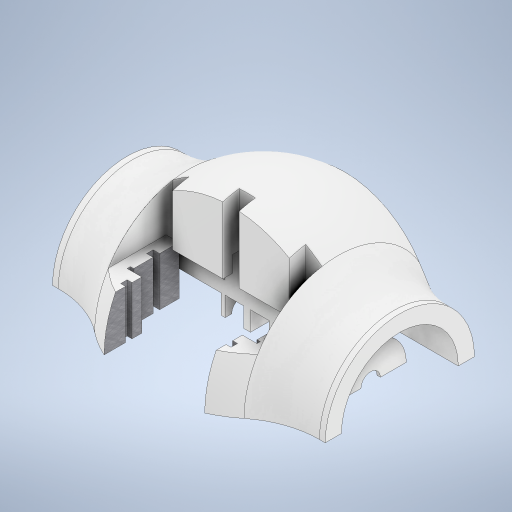
# Autodesk Inventor part: back moter middle tire lemon shape
Saved by Autodesk Inventor 2023 (Build 270158000, 158)
## iProperties
Created: 2022-10-08
Part Number: back moter middle tire lemon shape
Material: ABS プラスチック
Document SubType Name: Modeling
Designer: ellie
Density: 1.06 g/cm^3
Appearance: 積雪
Author: ellie
Autodesk Inventor part; units mm, degrees
ref_plane "YZ Plane" through (0, 0, 0) normal (1, 0, 0) x (0, 1, 0)
ref_plane "XZ Plane" through (0, 0, 0) normal (0, 1, 0) x (-1, 0, 0)
ref_plane "XY Plane" through (0, 0, 0) normal (0, 0, 1) x (1, 0, 0)
sketch "スケッチ1" plane through (0, 0, 0) normal (0, 1, 0) x (-1, 0, 0)
  circle A0 centre (0, 0) radius 37
  line L0 (0, 0) -> (0, -37)
  line L1 (0, 0) -> (0, 37)
  dimension "d0" = 74
  constraints: 4 end point, 2 point on circle, 2 vertical, 1 centre point, 1 coincident
  measures "d0" diameter of A0
revolve "回転1" add sketch "スケッチ1" angle 180 about axis through (0, 0, 0) along (0, 0, 1) picked at (-2.7444, -24.3574) contours L1 L0 A0
sketch "スケッチ5" plane through (0, 0, 0) normal (0, -1, 0) x (1, 0, 0)
  line L0 (-20, -21) -> (20, -21)
  line L1 (20, -21) -> (20, -11)
  line L2 (20, -11) -> (-20, -11)
  line L3 (-20, -11) -> (-20, -21)
  line L4 (-20, -13) -> (-20, -11)
  line L5 (0, 27) -> (-17, 27)
  line L6 (-17, 27) -> (-17, 25)
  line L7 (-17, 25) -> (0, 25)
  line L8 (0, 25) -> (0, 27)
  line L9 (0, 22) -> (-20, 22)
  line L10 (-20, 22) -> (-20, 21)
  line L11 (-20, 21) -> (0, 21)
  line L12 (0, 21) -> (0, 22)
  line L13 (0, 15) -> (-21, 15)
  line L14 (-21, 15) -> (-21, 13)
  line L15 (-21, 13) -> (0, 13)
  line L16 (0, 13) -> (0, 15)
  line L17 (0, 7) -> (-23, 7)
  line L18 (-23, 7) -> (-23, 5)
  line L19 (-23, 5) -> (0, 5)
  line L20 (0, 5) -> (0, 7)
  circle A0 centre (0, 0) radius 37 projected
  circle A1 centre (0, 0) radius 37 projected
  line L21 (0, 37) -> (0, -37)
  line L22 (37, 0) -> (-37, 0)
  line L23 (-32, 5) -> (-23, 5)
  line L24 (-23, 5) -> (-23, -5)
  line L25 (-23, -5) -> (-32, -5)
  line L26 (-32, -5) -> (-32, 5)
  line L27 (-23, -8.0262) -> (-23, 5)
  line L28 (-29, 22.9783) -> (-29, -22.9783)
  line L29 (-15.5, 27) -> (0, 27)
  line L30 (0, 27) -> (0, 37)
  line L31 (0, 37) -> (-15.5, 37)
  line L32 (-15.5, 37) -> (-15.5, 27)
  line L33 (-15.5, 25) -> (0, 25)
  line L34 (0, 25) -> (0, 22)
  line L35 (0, 22) -> (-15.5, 22)
  line L36 (-15.5, 22) -> (-15.5, 25)
  line L37 (-19, 15) -> (0, 15)
  line L38 (0, 15) -> (0, 21)
  line L39 (0, 21) -> (-19, 21)
  line L40 (-19, 21) -> (-19, 15)
  line L41 (-19, 13) -> (0, 13)
  line L42 (0, 13) -> (0, 7)
  line L43 (0, 7) -> (-19, 7)
  line L44 (-19, 7) -> (-19, 13)
  line L45 (-23, 0) -> (-39.6865, 0)
  line L46 (-23, 0) -> (-7.8337, 0)
  line L47 (-8, 5) -> (-23, 5)
  line L48 (-23, 5) -> (-23, -5)
  line L49 (-23, -5) -> (-8, -5)
  line L50 (-8, -5) -> (-8, 5)
  line L51 (-8, 5) -> (-23, -5) construction
  line L52 (-23, 5) -> (-8, -5) construction
  line L53 (-23, 7) -> (-33, 7)
  line L54 (-33, 7) -> (-33, -7)
  line L55 (-33, -7) -> (-23, -7)
  line L56 (-23, -7) -> (-23, 7)
  line L57 (-23, 7) -> (-33, -7) construction
  line L58 (-33, 7) -> (-23, -7) construction
  line L59 (-8, 5) -> (-1, 5)
  line L60 (-1, 5) -> (-1, -5)
  line L61 (-1, -5) -> (-8, -5)
  line L62 (-8, -5) -> (-8, 5)
  line L63 (-8, 5) -> (-1, -5) construction
  line L64 (-1, 5) -> (-8, -5) construction
  line L65 (-23, 5) -> (-29, 5)
  line L66 (-23, -5) -> (-29, -5)
  line L67 (-23, 7) -> (-29, 7)
  line L68 (-23, -7) -> (-29, -7)
  line L69 (27.2764, -25) -> (-27.2764, -25)
  line L70 (-8, 5) -> (-6.8, 5)
  line L71 (-6.8, 5) -> (-6.8, -5)
  line L72 (-6.8, -5) -> (-8, -5)
  line L73 (-8, -5) -> (-8, 5)
  line L74 (-3, 7) -> (0, 7)
  line L75 (0, 22) -> (-4, 22)
  line L76 (-4, 21) -> (0, 21)
  line L77 (0, 21) -> (0, 22)
  line L78 (-6, 7) -> (-1, 7)
  line L79 (-1, 5) -> (-6, 5)
  point P0 (0, -21)
  point P1 (0, -11)
  point P2 (0, 26)
  point P3 (0, 21.5)
  point P4 (0, 14)
  point P5 (0, 6)
  point P6 (-20, -16)
  point P7 (-27, -0.5262)
  point P8 (-29, -5)
  point P9 (-15.5, 23.5)
  point P10 (-15.5, 33.5969)
  point P11 (0, 27)
  point P12 (0, 25)
  point P13 (0, 13)
  point P14 (0, 15)
  point P15 (-29, 0)
  point P16 (-32, 0)
  point P17 (-23, 0)
  point P18 (-15.5, 0)
  point P19 (-28, 0)
  point P20 (-4.5, 0)
  point P21 (-8, -5)
  point P22 (-8, 5)
  point P23 (-27, 0.5)
  point P24 (-28, 0.4738)
  point P25 (-28, -11.5262)
  point P26 (-27, -11.5)
  point P27 (-23, -5)
  point P28 (-23, 5)
  point P29 (-23, 5)
  point P30 (-23, -5)
  point P31 (-8, 0)
  point P32 (-1, 0)
  point P33 (0, 21)
  point P34 (0, 22)
  point P35 (-29, -7)
  point P36 (-29, 7)
  dimension "d12" = 40
  dimension "d13" = 10
  dimension "d23" = 17
  dimension "d24" = 2
  dimension "d27" = 20
  dimension "d28" = 1
  dimension "d30" = 21
  dimension "d31" = 2
  dimension "d33" = 2
  dimension "d88" = 0
  dimension "d89" = 0
  dimension "d90" = 16
  dimension "d92" = 20
  dimension "d93" = 10
  dimension "d97" = 9
  dimension "d98" = 10
  dimension "d113" = 29
  dimension "d122" = 15.5
  dimension "d123" = 37
  dimension "d124" = 3
  dimension "d125" = 15.5
  dimension "d126" = 6
  dimension "d127" = 6
  dimension "d128" = 19
  dimension "d129" = 19
  dimension "d147" = 10
  dimension "d149" = 8
  dimension "d151" = 15
  dimension "d161" = 14
  dimension "d162" = 10
  dimension "d164" = 10
  dimension "d165" = 7
  dimension "d170" = 25
  dimension "d175" = 1.2
  dimension "d207" = 0
  constraints: 158 end point, 31 parallel, 20 horizontal, 17 perpendicular, 16 point on line, 15 midpoint, 10 collinear, 1 vertical, 20 other
  measures "d12" distance of L2.end L1.end
  measures "d13" distance of L1.end L0.end
  measures "d23" distance of L7.end L6.end
  measures "d24" distance of L6.end L5.end
  measures "d27" distance of L11.end L10.end
  measures "d28" distance of L10.end L9.end
  measures "d30" distance of L15.end L14.end
  measures "d31" distance of L14.end L13.end
  measures "d33" distance of L18.end L17.end
  measures "d89" distance from line of point (0, 0) L22
  measures "d90" distance from line of L0 point (0, -37)
  measures "d92" distance of the line from the sketch origin of L3
  measures "d93" distance from line of L5 point (0, 37)
  measures "d97" distance of L24.end L25.end
  measures "d98" distance of L23.end L24.end
  measures "d113" distance of the line from the sketch origin of L28
  measures "d122" distance of the line from the sketch origin of L32
  measures "d123" distance between parallel lines of L31 L22
  measures "d124" distance of L33.end L34.end
  measures "d126" distance of L38.end L37.end
  measures "d127" distance of L41.end L42.end
  measures "d128" distance of the line from the sketch origin of L44
  measures "d129" distance of the line from the sketch origin of L40
  measures "d147" distance of L48.end L47.end
  measures "d149" distance of the line from the sketch origin of L50
  measures "d151" distance between parallel lines of L50 L24
  measures "d161" distance between parallel lines of L55 L53
  measures "d162" distance between parallel lines of L48 L54
  measures "d164" distance between parallel lines of L61 L59
  measures "d165" distance between parallel lines of L50 L60
  measures "d170" distance between parallel lines of L69 L22
  measures "d175" distance of L71.end L72.end
  measures "d207" distance between parallel lines of L47 L19
extrude "GNSボード" cut sketch "スケッチ5" against normal blind 16 contours L8 L7 L6 L5
extrude "GNSボード止めるよう" cut sketch "スケッチ5" against normal blind 15 contours L21 L5 L32 A0 | L21 L9 L36 L7
extrude "アルミ板１" cut sketch "スケッチ5" against normal blind 20 contours L11 L10 L9 L12
extrude "メイン基板" cut sketch "スケッチ5" against normal blind 21 contours L15 L14 L13 L16
extrude "メイン止めるよう" cut sketch "スケッチ5" against normal blind 15 contours L17 L44 L15 L21 | L13 L40 L11 L21
extrude "アルミ板２" cut sketch "スケッチ5" against normal blind 20 contours L19 L18 L17 L20
extrude "電池ボックス入れ" cut sketch "スケッチ5" against normal blind 13 contours L3 L2 L21 L0 | L21 L2 L1 L0
extrude "side ut" cut sketch "スケッチ5" against normal blind 100 contours A0 L22 L54 L55 L28 | A0 L28 L53 L54 L22 | L55 L54 L22 L26 L25 L28 | L54 L53 L28 L23 L26 L22 | L25 L26 L22 L28 | L26 L23 L28 L22
extrude "motor case" add sketch "スケッチ5" against normal blind 7 contours L55 L54 L22 L26 L25 L28 | L28 L25 L27 L55 | L54 L53 L28 L23 L26 L22 | L28 L22 L24 L25 | L25 L26 L22 L28 | L50 L49 L24 L22 | L22 L24 L19 L50 | L53 L18 L23 L28 | L26 L23 L28 L22 | L28 L23 L24 L22
extrude "bottom cut" cut sketch "スケッチ5" against normal blind 90 contours L69 A0 L21 | L21 A0 L69
extrude "motor" cut sketch "スケッチ5" against normal blind 6 contours L60 L61 L71 L22 | L22 L71 L19 L60 | L71 L61 L50 L22 | L22 L50 L19 L71 | L28 L22 L24 L25 | L25 L26 L22 L28 | L50 L49 L24 L22 | L22 L24 L19 L50 | L26 L23 L28 L22 | L28 L23 L24 L22
extrude "motor block" add sketch "スケッチ5" against normal blind 10 contours L71 L61 L50 L22 | L22 L50 L19 L71
sketch "スケッチ27" plane through (-33, 0, -7) normal (-1, 0, 0) x (0, 0, 1)
  line L0 (14, 0) -> (0, 0) projected
  circle A0 centre (7, 0) radius 3
  point P0 (7, 0)
  dimension "d198" = 6
  constraints: 1 centre point, 1 midpoint
  measures "d198" diameter of A0
extrude "moter shaft" cut sketch "スケッチ27" against normal blind 27
mirror "ミラー13" about plane through (0, 0, 0) normal (1, 0, 0) of "メイン止めるよう", "メイン基板", "アルミ板１", "GNSボード止めるよう", "GNSボード", "アルミ板２", "motor", "motor case", "moter shaft", "電池ボックス入れ", "side ut", "motor block"
ref_plane "作業平面5" through (-17, 17.5, 25) normal (0, -1, 0) x (1, 0, 0)
ref_plane "作業平面6" through (20, 13, -11) normal (0, 0, -1) x (1, 0, 0)
ref_plane "作業平面7" through (29, 35, 7) normal (0, -1, 0) x (1, 0, 0)
sketch "スケッチ41" plane through (-17, 0, 25) normal (0, -1, 0) x (1, 0, 0)
  line L0 (-16, -22) -> (-15, -22) projected
  line L1 (-15, -22) -> (-15, -20) projected
  line L2 (-15, -20) -> (-6, -20) projected
  line L3 (-6, -20) -> (-6, -18) projected
  line L4 (-6, -18) -> (-2, -18) projected
  line L5 (-2, -18) -> (-2, -12) projected
  line L6 (-2, -12) -> (-4, -12) projected
  line L7 (-4, -12) -> (-4, -10) projected
  line L8 (-4, -10) -> (-2, -10) projected
  line L9 (-2, -10) -> (-2, -4) projected
  line L10 (-2, -4) -> (-3, -4) projected
  line L11 (-3, -4) -> (-3, -3) projected
  line L12 (-3, -3) -> (1.5, -3) projected
  line L13 (1.5, -3) -> (1.5, 0) projected
  line L14 (1.5, 0) -> (0, 0) projected
  line L15 (0, 0) -> (0, 2) projected
  line L16 (0, 2) -> (1.5, 2) projected
  line L17 (1.5, 2) -> (1.5, 8.5969) projected
  arc A0 (1.5, 8.5969) -> (-12, -2.0217) centre (17, -25) ccw projected
  line L18 (-12, -2.0217) -> (-12, -18) projected
  line L19 (-12, -18) -> (-16, -18) projected
  line L20 (-16, -18) -> (-16, -22) projected
  line L21 (-2, -18) -> (-2, -12) projected
  line L22 (-4, -10) -> (-4, -12) projected
  line L23 (0, 2) -> (0, 0) projected
  circle A1 centre (-4, 0.5) radius 2.4
  dimension "d252" = 4.8
  dimension "d253" = 4
  dimension "d254" = 3.5
  constraints: 1 centre point
  measures "d252" diameter of A1
  measures "d253" distance from line of A1.centre L15
  measures "d254" distance from line of A1.centre L12
extrude "top lock 10mm" cut sketch "スケッチ41" against normal blind 3 contours A1
mirror "ミラー15" about plane through (0, 0, 0) normal (1, 0, 0) of "top lock 10mm"
sketch "スケッチ42" plane through (-33, 0, -7) normal (0, -1, 0) x (1, 0, 0)
  circle A0 centre (9, -14.5) radius 2.4
  line L0 (13, -14) -> (13, -4) projected
  line L1 (32, 2) -> (1, 2) projected
  point P0 (33, 7)
  point P1 (10, 2)
  point P2 (6.8183, 2)
  point P3 (11.1817, 2)
  dimension "d257" = 4
  dimension "d258" = 4.8
  dimension "d259" = 16.5
  constraints: 1 centre point
  measures "d257" distance from line of A0.centre L0
  measures "d258" diameter of A0
  measures "d259" distance from line of A0.centre L1
extrude "bottom lock" cut sketch "スケッチ42" against normal blind 3
mirror "ミラー16" about plane through (0, 0, 0) normal (1, 0, 0) of "bottom lock"
ref_plane "作業平面8" through (-17, 15, 25) normal (0, -1, 0) x (1, 0, 0)
sketch "スケッチ45" plane through (-17, 15, 25) normal (0, -1, 0) x (1, 0, 0)
  circle A0 centre (-4, 0.5) radius 2.4 projected
  line L0 (-16, -22) -> (-15, -22) projected
  line L1 (-15, -22) -> (-15, -20) projected
  line L2 (-15, -20) -> (-6, -20) projected
  line L3 (-6, -20) -> (-6, -18) projected
  line L4 (-6, -18) -> (-2, -18) projected
  line L5 (-2, -18) -> (-2, -12) projected
  line L6 (-2, -12) -> (-4, -12) projected
  line L7 (-4, -12) -> (-4, -10) projected
  line L8 (-4, -10) -> (-2, -10) projected
  line L9 (-2, -10) -> (-2, -4) projected
  line L10 (-2, -4) -> (-3, -4) projected
  line L11 (-3, -4) -> (-3, -3) projected
  line L12 (-3, -3) -> (1.5, -3) projected
  line L13 (1.5, -3) -> (1.5, 0) projected
  line L14 (1.5, 0) -> (0, 0) projected
  line L15 (0, 0) -> (0, 2) projected
  line L16 (0, 2) -> (1.5, 2) projected
  line L17 (1.5, 2) -> (1.5, 8.5969) projected
  arc A1 (1.5, 8.5969) -> (-12, -2.0217) centre (17, -25) ccw projected
  line L18 (-12, -2.0217) -> (-12, -18) projected
  line L19 (-12, -18) -> (-16, -18) projected
  line L20 (-16, -18) -> (-16, -22) projected
  arc A2 (32.5, 5.0624) -> (1.5, 5.0624) centre (17, -25) ccw projected
  line L21 (1.5, 2) -> (1.5, 5.0624) projected
  line L22 (32.5, 2) -> (1.5, 2) projected
  line L23 (32.5, 2) -> (32.5, 5.0624) projected
  circle A3 centre (38, 0.5) radius 2.4 projected
  line L24 (49, -22) -> (50, -22) projected
  line L25 (50, -18) -> (50, -22) projected
  line L26 (46, -18) -> (50, -18) projected
  line L27 (46, -18) -> (46, -2.0217) projected
  arc A4 (46, -2.0217) -> (32.5, 8.5969) centre (17, -25) ccw projected
  line L28 (32.5, 8.5969) -> (32.5, 2) projected
  line L29 (32.5, 2) -> (34, 2) projected
  line L30 (34, 2) -> (34, 0) projected
  line L31 (34, 0) -> (32.5, 0) projected
  line L32 (32.5, 0) -> (32.5, -3) projected
  line L33 (32.5, -3) -> (37, -3) projected
  line L34 (37, -3) -> (37, -4) projected
  line L35 (37, -4) -> (36, -4) projected
  line L36 (36, -4) -> (36, -10) projected
  line L37 (36, -10) -> (38, -10) projected
  line L38 (38, -10) -> (38, -12) projected
  line L39 (38, -12) -> (36, -12) projected
  line L40 (36, -12) -> (36, -18) projected
  line L41 (36, -18) -> (40, -18) projected
  line L42 (40, -18) -> (40, -20) projected
  line L43 (40, -20) -> (49, -20) projected
  line L44 (49, -20) -> (49, -22) projected
  circle A5 centre (38, 0.5) radius 2.4 projected
  circle A6 centre (-4, 0.5) radius 2.4 projected
  line L45 (34, 0) -> (0, 0) projected
  line L46 (34, 0) -> (34, 2) projected
  line L47 (34, 2) -> (0, 2) projected
  line L48 (0, 0) -> (0, 2) projected
  line L49 (32.5, -3) -> (1.5, -3) projected
  line L50 (32.5, -3) -> (32.5, 0) projected
  line L51 (1.5, 0) -> (32.5, 0) projected
  line L52 (1.5, -3) -> (1.5, 0) projected
  line L53 (-2, -4) -> (36, -4) projected
  circle A7 centre (38, 0.5) radius 2.4 projected
  line L54 (36, -10) -> (-2, -10) projected
  line L55 (36, -10) -> (36, -4) projected
  line L56 (-2, -4) -> (36, -4) projected
  line L57 (-2, -10) -> (-2, -4) projected
  line L58 (-2, -12) -> (36, -12) projected
  line L59 (36, -18) -> (-2, -18) projected
  line L60 (36, -18) -> (36, -12) projected
  line L61 (-2, -12) -> (36, -12) projected
  line L62 (-2, -18) -> (-2, -12) projected
  line L63 (40, -20) -> (-6, -20) projected
  line L64 (40, -20) -> (40, -18) projected
  line L65 (40, -18) -> (-6, -18) projected
  line L66 (-6, -20) -> (-6, -18) projected
  line L67 (9, -30) -> (9, -20) projected
  line L68 (-6, -20) -> (9, -20) projected
  line L69 (-15, -20) -> (-6, -20) projected
  line L70 (-15, -30) -> (-15, -20) projected
  line L71 (16, -30) -> (10.2, -30) projected
  circle A8 centre (41, -46.5) radius 2.4 projected
  circle A9 centre (-7, -46.5) radius 2.4 projected
  line L72 (25, -28) -> (23.8, -28) projected
  line L73 (23.8, -30) -> (23.8, -28) projected
  line L74 (18, -30) -> (18, -20) projected
  line L75 (18, -20) -> (16, -20) projected
  line L76 (16, -20) -> (16, -30) projected
  line L77 (10.2, -30) -> (10.2, -28) projected
  line L78 (10.2, -28) -> (9, -28) projected
  line L79 (9, -20) -> (9, -22) projected
  line L80 (-6, -20) -> (-6, -18) projected
  line L81 (16, -30) -> (10.2, -30) projected
  line L82 (-15, -30) -> (-15, -28) projected
  line L83 (-15, -28) -> (-16, -28) projected
  line L84 (-16, -28) -> (-16, -32) projected
  line L85 (-16, -32) -> (-12, -32) projected
  line L86 (-12, -32) -> (-12, -47.9783) projected
  arc A10 (-12, -47.9783) -> (-10.2764, -50) centre (17, -25) ccw projected
  line L87 (-10.2764, -50) -> (44.2764, -50) projected
  arc A11 (44.2764, -50) -> (46, -47.9783) centre (17, -25) ccw projected
  line L88 (46, -47.9783) -> (46, -32) projected
  line L89 (50, -32) -> (46, -32) projected
  line L90 (50, -28) -> (50, -32) projected
  line L91 (50, -28) -> (49, -28) projected
  line L92 (49, -28) -> (49, -30) projected
  line L93 (23.8, -30) -> (18, -30) projected
  line L94 (40, -18) -> (40, -20) projected
  line L95 (25, -20) -> (25, -22) projected
  line L96 (-3, -36) -> (37, -36) projected
  line L97 (37, -36) -> (37, -46) projected
  line L98 (37, -46) -> (-3, -46) projected
  line L99 (-3, -46) -> (-3, -36) projected
  line L100 (-6, -15) -> (40, -15)
  line L101 (40, -15) -> (40, 8.8231)
  line L102 (40, 8.8231) -> (-6, 8.8231)
  line L103 (-6, 8.8231) -> (-6, -15)
  line L104 (10.2, -20) -> (10.2, -30) projected
  line L105 (16, -20) -> (16, -30) projected
  line L106 (10.2, -20) -> (16, -20) projected
  line L107 (9, -30) -> (-15, -30) projected
  line L108 (-16, -22) -> (-15, -22) projected
  line L109 (-15, -22) -> (-15, -20) projected
  line L110 (-15, -20) -> (-6, -20) projected
  line L111 (-6, -18) -> (-2, -18) projected
  line L112 (-2, -18) -> (-2, -12) projected
  line L113 (-2, -12) -> (-4, -12) projected
  line L114 (-4, -12) -> (-4, -10) projected
  line L115 (-4, -10) -> (-2, -10) projected
  line L116 (-2, -10) -> (-2, -4) projected
  line L117 (-2, -4) -> (-3, -4) projected
  line L118 (-3, -4) -> (-3, -3) projected
  line L119 (-3, -3) -> (1.5, -3) projected
  line L120 (1.5, -3) -> (1.5, 0) projected
  line L121 (1.5, 0) -> (0, 0) projected
  line L122 (0, 0) -> (0, 2) projected
  line L123 (0, 2) -> (1.5, 2) projected
  line L124 (1.5, 2) -> (1.5, 8.5969) projected
  line L125 (-12, -2.0217) -> (-12, -18) projected
  line L126 (-12, -18) -> (-16, -18) projected
  line L127 (-16, -18) -> (-16, -22) projected
  line L128 (9, -22) -> (10.2, -22) projected
  line L129 (10.2, -22) -> (10.2, -20) projected
  line L130 (10.2, -20) -> (9, -20) projected
  line L131 (9, -28) -> (9, -30) projected
  line L132 (9, -30) -> (-15, -30) projected
  line L133 (49, -30) -> (25, -30) projected
  line L134 (25, -28) -> (25, -30) projected
  line L135 (23.8, -22) -> (25, -22) projected
  line L136 (23.8, -20) -> (25, -20) projected
  line L137 (23.8, -22) -> (23.8, -20) projected
  line L138 (49, -22) -> (50, -22) projected
  line L139 (50, -18) -> (50, -22) projected
  line L140 (46, -18) -> (50, -18) projected
  line L141 (46, -18) -> (46, -2.0217) projected
  line L142 (32.5, 8.5969) -> (32.5, 2) projected
  line L143 (32.5, 2) -> (34, 2) projected
  line L144 (34, 2) -> (34, 0) projected
  line L145 (34, 0) -> (32.5, 0) projected
  line L146 (32.5, 0) -> (32.5, -3) projected
  line L147 (32.5, -3) -> (37, -3) projected
  line L148 (37, -3) -> (37, -4) projected
  line L149 (37, -4) -> (36, -4) projected
  line L150 (36, -4) -> (36, -10) projected
  line L151 (36, -10) -> (38, -10) projected
  line L152 (38, -10) -> (38, -12) projected
  line L153 (38, -12) -> (36, -12) projected
  line L154 (36, -12) -> (36, -18) projected
  line L155 (36, -18) -> (40, -18) projected
  line L156 (40, -20) -> (49, -20) projected
  line L157 (49, -20) -> (49, -22) projected
  arc A12 (1.5, 8.5969) -> (-12, -2.0217) centre (17, -25) ccw projected
  arc A13 (46, -2.0217) -> (32.5, 8.5969) centre (17, -25) ccw projected
  dimension "d269" = 3
  constraints: 8 end point, 2 collinear, 2 parallel, 1 horizontal, 1 perpendicular, 1 tangent
  measures "d269" distance between parallel lines of L100 L65
extrude "back cut" cut sketch "スケッチ45" against normal blind 25 contours A0 L103 | A0 L103 A1 L17 L16 L15 L14 L13 L12 L11 L10 L9 L8 L7 L6 L5 L100 | L103 L102 A2 L17 A1 | L5 L58 L40 L100 | A2 L23 L22 L17 | L102 L101 A4 L28 A2 | L6 L7 L8 L54 L37 L38 L39 L58 | L40 L39 L38 L37 L36 L35 L34 L33 L32 L31 L30 L29 L23 L28 A4 L101 A3 L100 | L22 L29 L30 L31 L45 L14 L15 L16 | A3 L101 | L9 L53 L36 L54 | L45 L32 L49 L13 | L10 L11 L12 L49 L33 L34 L35 L53 picked at (-4.4805, 1.0136) picked at (38.5393, 0.5971)
sketch "スケッチ52" plane through (20, 0, -11) normal (0, 0, -1) x (-1, 0, 0)
  line L0 (40, 0) -> (0, 0) projected
  line L1 (40, 0) -> (40, 13) projected
  line L2 (40, 13) -> (0, 13) projected
  line L3 (0, 0) -> (0, 13) projected
  line L4 (28, 0) -> (28, 6) projected
  line L5 (28, 6) -> (52, 6) projected
  line L6 (52, 0) -> (52, 6) projected
  line L7 (28, 0) -> (52, 0) projected
  line L8 (26.8, 6) -> (26.8, 0) projected
  line L9 (21, 0) -> (26.8, 0) projected
  line L10 (21, 0) -> (21, 6) projected
  line L11 (21, 6) -> (26.8, 6) projected
  line L12 (13.2, 0) -> (13.2, 6) projected
  line L13 (19, 6) -> (13.2, 6) projected
  line L14 (19, 0) -> (19, 6) projected
  line L15 (13.2, 0) -> (19, 0) projected
  line L16 (12, 6) -> (12, 0) projected
  line L17 (-12, 0) -> (12, 0) projected
  line L18 (-12, 0) -> (-12, 6) projected
  line L19 (12, 6) -> (-12, 6) projected
  line L20 (27, 10) -> (37, 10)
  line L21 (37, 10) -> (37, 16)
  line L22 (37, 16) -> (27, 16)
  line L23 (27, 16) -> (27, 10)
  point P0 (20, 0)
  dimension "d293" = 3
  dimension "d294" = 10
  dimension "d295" = 4
  constraints: 8 end point, 2 parallel, 1 horizontal, 1 perpendicular, 1 other
  measures "d293" distance between parallel lines of L1 L21
  measures "d294" distance between parallel lines of L21 L23
  measures "d295" distance between parallel lines of L20 L5
extrude "押し出し54" cut sketch "スケッチ52" against normal up to surface (18 mm away) contours L21 L20 L23 L2 | L2 L23 L22 L21
sketch "スケッチ53" plane through (0, 13, 0) normal (0, -1, 0) x (1, 0, 0)
  line L0 (-7, -11) -> (-7, 5) projected
  line L1 (-17, -11) -> (-7, -11) projected
  line L2 (-17, -11) -> (-17, 5) projected
  line L3 (-17, -11) -> (-17, 5) projected
  line L4 (-17, -11) -> (-17, 5) projected
  line L5 (-23, 10) -> (23, 10) projected
  line L6 (23, 10) -> (23, 24.7992) projected
  arc A0 (23, 24.7992) -> (15.5, 30.0624) centre (0, 0) ccw projected
  line L7 (15.5, 30.0624) -> (15.5, 33.5969) projected
  arc A1 (29, 22.9783) -> (15.5, 33.5969) centre (0, 0) ccw projected
  line L8 (29, 22.9783) -> (29, -22.9783) projected
  line L9 (27.2764, -25) -> (-27.2764, -25) projected
  arc A2 (-29, -22.9783) -> (-27.2764, -25) centre (0, 0) ccw projected
  line L10 (-29, -22.9783) -> (-29, 22.9783) projected
  line L11 (-15.5, 33.5969) -> (-15.5, 30.0624) projected
  arc A3 (-15.5, 30.0624) -> (-23, 24.7992) centre (0, 0) ccw projected
  line L12 (-23, 24.7992) -> (-23, 10) projected
  line L13 (-17, -11) -> (-7, -11)
  line L14 (-7, -11) -> (-7, -17)
  line L15 (-7, -17) -> (-17, -17)
  line L16 (-17, -17) -> (-17, -11)
  arc A4 (27.2764, -25) -> (29, -22.9783) centre (0, 0) ccw projected
  arc A5 (-15.5, 33.5969) -> (-29, 22.9783) centre (0, 0) ccw projected
  point P0 (-17, -11)
  point P1 (-7, -11)
  dimension "d298" = 6
  constraints: 8 end point, 3 collinear, 2 parallel, 1 horizontal, 1 perpendicular
  measures "d298" distance between parallel lines of L15 L1
extrude "押し出し55" cut sketch "スケッチ53" against normal up to surface (3 mm away) contours L1 L14 L15 L16
sketch "スケッチ54" plane through (-23, 15, 10) normal (0, 0, 1) x (1, 0, 0)
  line L0 (42, 0) -> (46, 0) projected
  line L1 (46, 0) -> (41, 0)
  line L2 (41, 0) -> (41, 22)
  line L3 (41, 22) -> (46, 22)
  line L4 (46, 22) -> (46, 0)
  line L5 (0, 0) -> (4, 0) projected
  line L6 (0, 0) -> (5, 0)
  line L7 (5, 0) -> (5, 22)
  line L8 (5, 22) -> (0, 22)
  line L9 (0, 22) -> (0, 0)
  line L10 (23, -15) -> (23, 22)
  arc A0 (52, 7.9783) -> (-6, 7.9783) centre (23, -15) ccw projected
  line L11 (25.5, 0) -> (20.5, 0)
  line L12 (20.5, 0) -> (20.5, 22)
  line L13 (20.5, 22) -> (25.5, 22)
  line L14 (25.5, 22) -> (25.5, 0)
  line L15 (42, 0) -> (4, 0) projected
  arc A1 (46, 12.2029) -> (0, 12.2029) centre (23, -15) ccw projected
  line L16 (0, 0) -> (0, 12.2029) projected
  line L17 (0, 0) -> (4, 0) projected
  line L18 (42, 0) -> (4, 0) projected
  line L19 (42, 0) -> (46, 0) projected
  line L20 (46, 0) -> (46, 12.2029) projected
  line L21 (46, 0) -> (38.5, 0) projected
  line L22 (38.5, 0) -> (38.5, -15) projected
  line L23 (38.5, -15) -> (52, -15) projected
  line L24 (52, -15) -> (52, -15) projected
  arc A2 (50.2764, -15) -> (-4.2764, -15) centre (23, -15) ccw projected
  line L25 (-4.2764, -15) -> (-6, -15) projected
  line L26 (-6, -15) -> (-6, -15) projected
  line L27 (7.5, -15) -> (7.5, 0) projected
  line L28 (7.5, 0) -> (0, 0) projected
  line L29 (0, 0) -> (0, 12.2029) projected
  arc A3 (46, 12.2029) -> (0, 12.2029) centre (23, -15) ccw projected
  line L30 (46, 12.2029) -> (46, 0) projected
  line L31 (52, -15) -> (50.2764, -15) projected
  line L32 (-6, -15) -> (7.5, -15) projected
  point P0 (20.5, 0)
  point P1 (20.5, 21.9154)
  point P2 (5, 17.3265)
  point P3 (41, 17.3265)
  point P4 (25.5, 21.9154)
  point P5 (25.5, 0)
  point P6 (41, 15.7409)
  point P7 (25.5, 20.5352)
  point P8 (20.5, 20.5352)
  point P9 (5, 15.7409)
  point P10 (0, 12.2029)
  point P11 (4, 0)
  point P12 (46, 13.9828)
  point P13 (0, 13.9828)
  point P14 (4, 0)
  dimension "d301" = 5
  dimension "d302" = 5
  dimension "d303" = 2.5
  dimension "d304" = 5
  constraints: 26 end point, 6 parallel, 3 horizontal, 3 perpendicular, 3 tangent, 1 collinear, 1 point on circle, 1 vertical
  measures "d301" distance of L2.end L3.end
  measures "d302" distance of L8.end L7.end
  measures "d303" distance between parallel lines of L14 L10
  measures "d304" distance between parallel lines of L14 L12
extrude "押し出し56" cut sketch "スケッチ54" against normal up to surface (5 mm away) contours L1 L2 A2 L0 | A2 L2 A1 L4 L0 | A1 L2 A0 L4 | A2 L10 A1 L14 | L14 L11 L10 A2 | A0 L2 L3 L4 | A1 L10 A0 L14 | A2 L12 A1 L10 | L10 L11 L12 A2 | A0 L13 L14 | A1 L12 A0 L10 | A0 L12 L13 | A2 L5 L9 A1 L7 | L7 L6 L5 A2 | A1 L9 A0 L7
sketch "スケッチ55" plane through (-29, 0, 7) normal (-1, 0, 0) x (0, 0, 1)
  arc A0 (15.9783, 0) -> (-29.9783, 0) centre (-7, 0) ccw projected
  line L0 (-14, 7) -> (0, 7) projected
  line L1 (0, 0) -> (0, 7) projected
  line L2 (-14, 0) -> (-14, 7) projected
  arc A1 (-4, 0) -> (-10, 0) centre (-7, 0) ccw projected
  line L3 (-14, 0) -> (0, 0) projected
  line L4 (15.9783, 0) -> (0, 0) projected
  line L5 (-2, 0) -> (-12, 0) projected
  circle A2 centre (-7, 0) radius 11
  line L6 (-14, 0) -> (-29.9783, 0) projected
  point P0 (-31, 8)
  point P1 (-31, 0)
  point P2 (4, 0)
  point P3 (-18, 0)
  point P4 (-18, 0)
  dimension "d309" = 22
  constraints: 1 centre point, 1 coincident
  measures "d309" diameter of A2
extrude "モーター受け円形" add sketch "スケッチ55" along normal up to surface (4 mm away) contours L4 L1 L0 L2 L6 A2
sketch "スケッチ57" plane through (-29, 0, 0) normal (-1, 0, 0) x (0, 0, 1)
  circle A0 centre (0, 0) radius 16
  circle A1 centre (0, 0) radius 18
  line L0 (22.9783, 0) -> (11, 0) projected
  line L1 (-3, 0) -> (-11, 0) projected
  line L2 (11, 0) -> (3, 0) projected
  line L3 (5, 0) -> (-5, 0) projected
  arc A2 (3, 0) -> (-3, 0) centre (0, 0) ccw projected
  line L4 (11, 0) -> (3, 0) projected
  arc A3 (11, 0) -> (-11, 0) centre (0, 0) ccw projected
  line L5 (-3, 0) -> (-11, 0) projected
  arc A4 (11, 0) -> (-11, 0) centre (0, 0) ccw projected
  line L6 (22.9783, 0) -> (11, 0) projected
  arc A5 (22.9783, 0) -> (-22.9783, 0) centre (0, 0) ccw projected
  line L7 (-11, 0) -> (-22.9783, 0) projected
  point P0 (-16, 0)
  point P1 (11, 0)
  point P2 (16, 0)
  point P3 (-18, 0)
  point P4 (18, 0)
  dimension "d314" = 32
  dimension "d315" = 36
  constraints: 2 centre point, 2 coincident
  measures "d314" diameter of A0
  measures "d315" diameter of A1
extrude "押し出し59" cut sketch "スケッチ57" against normal blind 5 contours L0 A3 L7 A0
extrude "押し出し60" cut sketch "スケッチ57" against normal blind 5 contours A0 L7 A1 L0 picked at (-17.159, 1.4359)
mirror "ミラー17" about plane through (0, 0, 0) normal (1, 0, 0) of "モーター受け円形", "押し出し59", "押し出し60"
ref_plane "作業平面9" through (42, 0, 0) normal (1, 0, 0) x (0, 0, -1)
sketch "スケッチ59" plane through (42, 0, 0) normal (1, 0, 0) x (0, 0, -1)
  circle A0 centre (0, 0) radius 23
  arc A1 (18, 0) -> (-18, 0) centre (0, 0) ccw projected
  circle A2 centre (0, 0) radius 18
  line L0 (-22.9783, 0) -> (-33.5969, 0) projected
  line L1 (-18, 0) -> (-22.9783, 0) projected
  line L2 (-11, 0) -> (-18, 0) projected
  line L3 (-11, 0) -> (-3, 0) projected
  line L4 (5, 0) -> (-5, 0) projected
  line L5 (3, 0) -> (11, 0) projected
  line L6 (18, 0) -> (11, 0) projected
  line L7 (22.9783, 0) -> (18, 0) projected
  arc A3 (22.9783, 0) -> (-22.9783, 0) centre (0, 0) ccw projected
  line L8 (-22.9783, 0) -> (22.9783, 0)
  point P0 (17.6, 0)
  dimension "d321" = 46
  constraints: 2 centre point, 2 coincident, 2 end point, 1 concentric
  measures "d321" diameter of A0
extrude "押し出し61" add sketch "スケッチ59" against normal up to surface (13 mm away) contours A1 L1 A3 L7
sketch "スケッチ60" plane through (23, 0, 5) normal (0, -1, 0) x (1, 0, 0)
  point P0 (-23, -5)
fillet "面フィレット1" radius 27.7 1 edges at (29, 22.9783, 0)
mirror "ミラー18" about plane through (0, 0, 0) normal (1, 0, 0) of "面フィレット1", "押し出し61"
ref_plane "作業平面11" through (0, 13, 0) normal (0, -1, 0) x (1, 0, 0)
sketch "スケッチ61" plane through (0, 13, 0) normal (0, -1, 0) x (1, 0, 0)
  point P0 (0, 0)
